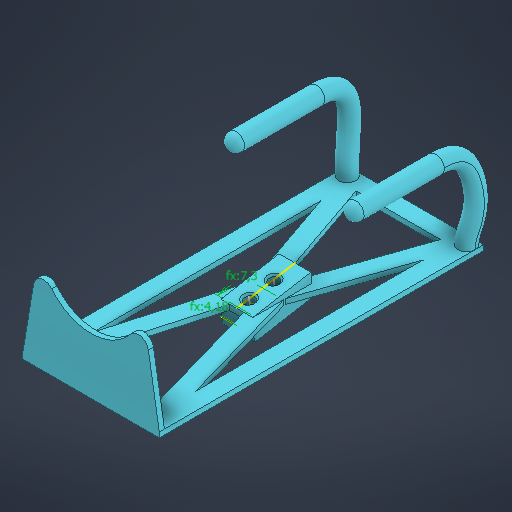
# Autodesk Inventor part: my_portafilter_holder_8
Saved by Autodesk Inventor 2026 (Build 300175000, 175)
## iProperties
Created: 2025-05-06
Part Number: my_portafilter_holder_8
Material: Generic
Document SubType Name: Modeling
Designer: Paul Juschitz
Density: 1 g/cm^3
Appearance: Cadet Blue
Author: Paul Juschitz
Autodesk Inventor part; units mm, degrees
ref_plane "YZ Plane" through (0, 0, 0) normal (1, 0, 0) x (0, 1, 0)
ref_plane "XZ Plane" through (0, 0, 0) normal (0, 1, 0) x (-1, 0, 0)
ref_plane "XY Plane" through (0, 0, 0) normal (0, 0, 1) x (1, 0, 0)
sketch "Sketch1" plane through (0, 0, 0) normal (0, 1, 0) x (-1, 0, 0)
  line L0 (20, 47.5) -> (-20, 47.5)
  line L1 (-20, 47.5) -> (-20, -47.5)
  line L2 (-20, -47.5) -> (20, -47.5)
  line L3 (20, -47.5) -> (20, 47.5)
  line L4 (20, 47.5) -> (-20, -47.5) construction
  line L5 (-20, 47.5) -> (20, -47.5) construction
  point P0 (0, 0)
  dimension "holder_width" = 40
  dimension "holder_length" = 95
  constraints: 12 end point, 2 midpoint, 2 parallel, 1 horizontal, 1 perpendicular
  measures "holder_width" distance of L2.end L1.end
  measures "holder_length" distance of L1.end L0.end
extrude "Extrusion1" add sketch "Sketch1" along normal blind 1.5
sketch "Sketch2" plane through (0, 1.5, 0) normal (0, 1, 0) x (1, 0, 0)
  line L0 (-20, 47.5) -> (-20, -47.5) projected
  line L1 (20, -47.5) -> (20, 47.5) projected
  line L2 (-20, -47.5) -> (20, -47.5)
  line L3 (20, -47.5) -> (20, -46)
  line L4 (20, -46) -> (-20, -46)
  line L5 (-20, -46) -> (-20, -47.5)
  point P0 (0, 0)
  point P1 (-20, -46)
  dimension "d4" = 1.5
  constraints: 8 end point, 2 parallel, 1 horizontal, 1 perpendicular, 1 point on line
  measures "d4" distance of L3.end L2.end
extrude "Extrusion2" add sketch "Sketch2" along normal blind 25
sketch "Sketch3" plane through (0, 1.5, 0) normal (0, 1, 0) x (1, 0, 0)
  circle A0 centre (17.5, 45) radius 2.5
  line L0 (20, 47.5) -> (-20, 47.5) projected
  line L1 (20, -46) -> (20, 47.5) projected
  point P0 (0, 0)
  dimension "prong_diameter" = 5
  constraints: 2 tangent, 1 centre point
  measures "prong_diameter" diameter of A0
sketch3d "3D Sketch1"
  spline S0 degree 4 poles (17.5, 1.5, -45) (17.5, 5.5, -45) (20, 9.5, -47.5) (17.5, 21.5, -47.5) (17.5, 26.5, -42) (17.5, 26.5, -36) knots 1 1 1 1 1 2 3 3 3 3 3
  line L0 (17.5, 26.5, -36) -> (17.5, 26.5, -10.0001)
  dimension "d14" = 35
  dimension "d15" = 8
  dimension "d16" = 20
  dimension "d17" = 6
  dimension "d18" = 9
  dimension "d19" = 4
  dimension "prong_height" = 25
  dimension "prong_length" = 34.9999
sweep "Sweep1" add profiles "Sketch3" path "3D Sketch1" contours A0
fillet "Fillet1" radius 2.5 1 edges at (15.0105, 26.2713, -10.0001)
mirror "Mirror1" about plane through (0, 0, 0) normal (1, 0, 0) of "Fillet1", "Sweep1"
sketch "Sketch5" plane through (0, 1.5, 0) normal (0, 1, 0) x (1, 0, 0)
  line L0 (17.5, 47.5) -> (-17.5, 47.5) construction
  line L1 (-20, 45) -> (-20, -46) construction
  line L2 (20, -46) -> (-20, -46) construction
  line L3 (20, -46) -> (20, 45) construction
  line L4 (20, 45) -> (20, 47.5) construction
  line L5 (20, 47.5) -> (17.5, 47.5) construction
  line L6 (-17.5, 47.5) -> (-20, 47.5) construction
  line L7 (-20, 47.5) -> (-20, 45) construction
  line L8 (-20, 47.5) -> (20, 47.5)
  line L9 (20, 47.5) -> (20, -46)
  line L10 (20, -46) -> (-20, -46)
  line L11 (-20, -46) -> (-20, 47.5)
  line L12 (-15, -41) -> (-15, 42.5) construction
  line L13 (-15, 42.5) -> (15, 42.5) construction
  line L14 (15, 42.5) -> (15, -41) construction
  line L15 (15, -41) -> (-15, -41) construction
  line L16 (0, 47.5) -> (0, -46)
  line L17 (-4.66, 12.5) -> (4.66, 12.5) construction
  line L18 (4.66, 12.5) -> (4.66, -4.8) construction
  line L19 (4.66, -4.8) -> (-4.66, -4.8) construction
  line L20 (-4.66, -4.8) -> (-4.66, 12.5) construction
  line L21 (-4.66, 12.5) -> (4.66, -4.8) construction
  line L22 (4.66, 12.5) -> (-4.66, -4.8) construction
  line L23 (15, 34.8279) -> (4.66, 4.8279)
  line L24 (12.3557, 42.5) -> (2.0157, 12.5)
  line L25 (15, 42.5) -> (4.66, 12.5) construction
  line L26 (15, -31.8975) -> (4.66, 4.3025)
  line L27 (12.4, -41) -> (2.06, -4.8)
  line L28 (15, -41) -> (4.66, -4.8) construction
  line L29 (-15, 34.8279) -> (-4.66, 4.8279)
  line L30 (-12.3557, 42.5) -> (-2.0157, 12.5)
  line L31 (-15, 42.5) -> (-4.66, 12.5) construction
  line L32 (-15, -31.8975) -> (-4.66, 4.3025)
  line L33 (-12.4, -41) -> (-2.06, -4.8)
  line L34 (-15, -41) -> (-4.66, -4.8) construction
  line L35 (-2.0157, 12.5) -> (2.0157, 12.5)
  line L36 (4.66, 4.8279) -> (4.66, 4.3025)
  line L37 (2.06, -4.8) -> (-2.06, -4.8)
  line L38 (-4.66, 4.8279) -> (-4.66, 4.3025)
  line L39 (-15, 34.8279) -> (-15, -31.8975)
  line L40 (-12.4, -41) -> (12.4, -41)
  line L41 (15, -31.8975) -> (15, 34.8279)
  line L42 (12.3557, 42.5) -> (-12.3557, 42.5)
  point P0 (0, 0)
  point P1 (0, 3.85)
  dimension "d34" = 5
  dimension "d35" = 9.32
  dimension "d36" = 17.3
  dimension "d37" = 35
  dimension "d38" = 5
  dimension "d39" = 5
  constraints: 70 end point, 9 point on line, 8 symmetric about line, 6 parallel, 4 collinear, 4 midpoint, 4 perpendicular, 3 horizontal, 1 vertical, 5 other
  measures "d34" distance between parallel lines of L1 L12
  measures "d35" distance of L18.end L19.end
  measures "d36" distance between parallel lines of L17 L19
  measures "d37" distance between parallel lines of L0 L17
  measures "d38" distance between parallel lines of L23 L24
  measures "d39" distance between parallel lines of L26 L27
extrude "Extrusion3" cut sketch "Sketch5" against normal up to surface (1.5 mm away) contours L42 L24 L35 L16 | L16 L35 L30 L42 | L40 L33 L37 L16 | L16 L37 L27 L40 | L41 L26 L36 L23 | L29 L38 L32 L39
sketch "Sketch8" plane through (-20, 0, 47.5) normal (0, 0, 1) x (1, 0, 0)
  arc A0 (8.5, 22.0557) -> (3.1867, 20.6595) centre (6.1499, 20.1911) ccw
  arc A1 (8.5, 22.0557) -> (31.5, 22.0557) centre (20, 31.18) ccw
  arc A2 (36.8095, 20.6833) -> (31.5, 22.0557) centre (33.8501, 20.1911) ccw
  line L0 (20, 0) -> (20, 47.7301)
  circle A3 centre (37.5, 26.5) radius 2.5 construction
  line L1 (20, 16.5) -> (37.5, 16.5) construction
  line L2 (37.5, 16.5) -> (37.5, 29) construction
  line L3 (0, 1.5) -> (40, 1.5) construction
  line L4 (40, 0) -> (40, 1.5) projected
  line L5 (40, 0) -> (40, 1.5)
  line L6 (40, 1.5) -> (36.8095, 20.6833)
  line L7 (0, 0) -> (0, 1.5)
  line L8 (0, 1.5) -> (3.1905, 20.6833)
  line L9 (0, 0) -> (0, 26.5) projected
  line L10 (0, 26.5) -> (40, 26.5) projected
  line L11 (40, 0) -> (40, 26.5) projected
  point P0 (3.1905, 20.6833)
  dimension "basket_handle_height" = 12.5
  dimension "d54" = 14.68
  dimension "d55" = 3
  dimension "d56" = 23
  constraints: 14 end point, 8 point on circle, 3 centre point, 3 tangent, 2 symmetric about line, 1 collinear, 1 equal radius, 1 horizontal, 1 line through centre, 1 perpendicular, 1 point on line, 1 vertical, 1 other
  measures "basket_handle_height" distance of L1.end L2.end
  measures "d54" radius of A1
  measures "d55" radius of A2
  measures "d56" distance of A1.end A0.start
extrude "Extrusion5" cut sketch "Sketch8" against normal up to surface (1.5 mm away)
sketch "Sketch9" plane through (0, 0, 0) normal (0, -1, 0) x (1, 0, 0)
  line L0 (4.66, 4.8) -> (-4.66, 4.8)
  line L1 (-4.66, 4.8) -> (-4.66, -12.5)
  line L2 (-4.66, -12.5) -> (4.66, -12.5)
  line L3 (4.66, -12.5) -> (4.66, 4.8)
  point P0 (0, 0)
  point P1 (2.06, 4.8)
  point P2 (-2.06, 4.8)
  point P3 (-4.66, -4.3025)
  point P4 (-4.66, -4.8279)
  point P5 (-2.0157, -12.5)
  point P6 (2.0157, -12.5)
  point P7 (4.66, -4.8279)
  point P8 (4.66, -4.3025)
  constraints: 8 end point, 4 point on line, 2 parallel, 1 horizontal, 1 perpendicular
extrude "Extrusion6" add sketch "Sketch9" along normal blind 0.1
sketch "Sketch10" plane through (0, -0.1, 0) normal (0, -1, 0) x (1, 0, 0)
  line L0 (-4.66, 4.8) -> (-4.66, -12.5) projected
  line L1 (-4.66, -12.5) -> (4.66, -12.5) projected
  line L2 (4.66, -12.5) -> (4.66, 4.8) projected
  line L3 (4.66, 4.8) -> (-4.66, 4.8) projected
  point P0 (0, 0)
revolve "Revolution1" add sketch "Sketch10" angle 10 about axis through (-4.66, -0.1, -12.5) along (1, 0, 0)
sketch "Sketch11" plane through (-4.66, -0.1, -12.5) normal (0, -0.9848078, -0.1736482) x (1, 0, 0)
  line L0 (0, 0) -> (9.32, 0) construction
  line L1 (4.66, 0) -> (4.66, 17.3)
  line L2 (9.32, 17.3) -> (0, 17.3) projected
  point P0 (4.66, 12.2927)
  point P1 (4.66, 5.82)
  point P2 (4.66, 13.12)
  point P3 (4.66, 17.3)
  dimension "d62" = 4.18
  dimension "d63" = 7.3
  constraints: 3 midpoint, 2 end point, 2 point on line, 1 vertical
  measures "d62" distance of point (4.66, 17.3) point (4.66, 13.12)
  measures "d63" distance of point (4.66, 5.82) point (4.66, 13.12)
sketch "Sketch13" plane through (0, 1.5, 0) normal (0, 1, 0) x (1, 0, 0)
  line L0 (4.66, -4.8) -> (4.66, 4.3025) projected
  line L1 (-2.0157, 12.5) -> (-4.66, 12.5) projected
  line L2 (4.66, -4.8) -> (-4.66, -4.8)
  line L3 (-4.66, -4.8) -> (-4.66, 12.5)
  line L4 (-4.66, 12.5) -> (4.66, 12.5)
  line L5 (4.66, 12.5) -> (4.66, -4.8)
  point P0 (0, 0)
  point P1 (2.06, -4.8)
  point P2 (2.0157, 12.5)
  point P3 (-4.66, 4.8279)
  constraints: 8 end point, 2 parallel, 1 horizontal, 1 perpendicular
revolve "Revolution2" add sketch "Sketch13" angle 10 about axis through (4.66, 1.5, 4.8) along (1, 0, 0)
sketch "Sketch14" plane through (0, 0, 0) normal (1, 0, 0) x (0, 1, 0)
  line L0 (-1.1106, -6.7684) -> (3.3996, -5.9731)
  line L1 (1.5, 4.8) -> (4.5041, -12.2372) projected
  line L2 (-2.3783, 0.4207) -> (2.7052, 1.317)
  line L3 (-0.1, -12.5) -> (-3.1041, 4.5372) projected
  point P0 (0, 0)
  constraints: 4 end point, 1 parallel, 1 perpendicular, 1 point on line
sketch "Sketch15" plane through (-4.66, 1.5, 4.8) normal (0, 0.9848078, 0.1736482) x (1, 0, 0)
  point P0 (4.66, 4.4666)
  point P1 (4.66, 3.6393)
  point P2 (4.66, 10.9393)
sketch "Sketch16" plane through (-4.66, -0.1, -12.5) normal (0, -0.9848078, -0.1736482) x (1, 0, 0)
  line L0 (0, 0) -> (9.32, 0) projected
  line L1 (9.32, 0) -> (9.32, 17.3) projected
  line L2 (9.32, 17.3) -> (0, 17.3) projected
  line L3 (0, 17.3) -> (0, 0) projected
  point P0 (4.66, 12.2927)
extrude "Extrusion7" add sketch "Sketch16" along normal blind 2
hole "Hole3" at (0, 2.132, 1.216) at (0, 3.3996, -5.9731) direction (0, -0.9848078, -0.1736482) diameter 3 end through all countersink diameter 4 countersink angle 90
equation "\"d4\" = print_thickness_1"
equation "\"d22\" = 0.5 * prong_diameter"
equation "\"d34\" = prong_diameter"
equation "\"d35\" = load_cell_width"
equation "\"d37\" = holder_load_cell_setback"
equation "\"d38\" = prong_diameter"
equation "\"d39\" = prong_diameter"
equation "\"d54\" = handle_radius"
equation "\"d62\" = load_cell_hole_inset"
equation "\"d63\" = load_cell_hole_spacing"
equation "\"d64\" = holder_angle"
equation "\"handle_circumference\" = 92.237"
equation "\"handle_radius\" = 0.159155 * handle_circumference"
equation "\"print_thickness_1\" = 1.5"
equation "\"load_cell_width\" = 9.32"
equation "\"holder_load_cell_setback\" = 35"
equation "\"holder_angle\" = 10deg"
equation "\"load_cell_hole_inset\" = 4.18"
equation "\"load_cell_hole_spacing\" = 7.3"
body "Solid1"
